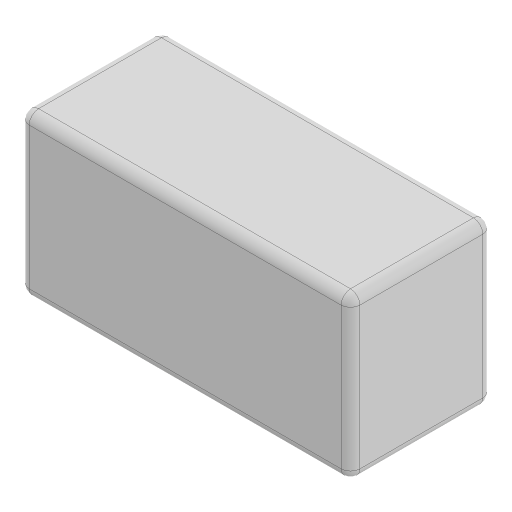
# Autodesk Inventor part: Battery Pack
Saved by Autodesk Inventor 2023 (Build 270158000, 158)
## iProperties
Created: 2022-03-03
Part Number: Battery Pack
Material: Generic
Document SubType Name: Modeling
Designer: Jochen
Density: 1 g/cm^3
Appearance: Default
Author: Jochen
Autodesk Inventor part; units mm, degrees
ref_plane "YZ Plane" through (0, 0, 0) normal (1, 0, 0) x (0, 1, 0)
ref_plane "XZ Plane" through (0, 0, 0) normal (0, 1, 0) x (-1, 0, 0)
ref_plane "XY Plane" through (0, 0, 0) normal (0, 0, 1) x (1, 0, 0)
sketch "Sketch1" plane through (0, 0, 0) normal (0, 0, 1) x (1, 0, 0)
  line L0 (0, -23.8) -> (0, 23.8) construction
  line L1 (-49, 0) -> (49, 0) construction
  line L2 (-35, -17) -> (35, -17)
  line L3 (35, -17) -> (35, 17)
  line L4 (35, 17) -> (-35, 17)
  line L5 (-35, 17) -> (-35, -17)
  line L6 (-35, -17) -> (35, 17) construction
  line L7 (35, -17) -> (-35, 17) construction
  point P0 (0, 0)
  dimension "d0" = 70
  dimension "d1" = 34
  constraints: 12 end point, 2 midpoint, 2 parallel, 1 horizontal, 1 perpendicular
  measures "d0" distance of L4.end L3.end
  measures "d1" distance of L4.end L2.start
extrude "Extrusion1" add sketch "Sketch1" along normal blind 30
fillet "Fillet1" radius 2 12 edges at (0, 17, 30) (0, 17, 0) (35, 17, 15) (35, 0, 30) (35, 0, 0) (35, -17, 15) (0, -17, 30) (-35, 0, 30) (-35, -17, 15) (-35, 0, 0) (0, -17, 0) (-35, 17, 15)
body "Solid1"
